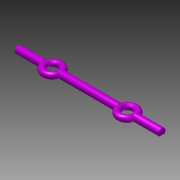
# Autodesk Inventor part: new string management system
Saved by Autodesk Inventor 2013 (Build 170138000, 138)
## iProperties
Created: 2014-03-08
Part Number: new string management system
Material: ABS Plastic
Document SubType Name: Modeling
Designer: kahohbein
Density: 1 g/cm^3
Author: kahohbein
Autodesk Inventor part; units mm, degrees
ref_plane "XZ Plane" through (0, 0, 0) normal (0, 1, 0) x (-1, 0, 0)
ref_plane "XY Plane" through (0, 0, 0) normal (0, 0, 1) x (1, 0, 0)
sketch "Sketch1" plane through (0, 0, 0) normal (0, 0, 1) x (1, 0, 0)
  line L0 (0, 0) -> (0, 6.5228)
  circle A0 centre (5, 0) radius 2
  dimension "d0" = 4
  dimension "d1" = 5
  constraints: 2 end point, 1 centre point, 1 vertical
  measures "d0" diameter of A0
  measures "d1" distance from line of A0.centre L0
revolve "Revolution1" add sketch "Sketch1" angle 360 about axis through (0, 0, 0) along (0, 1, 0)
ref_plane "Work Plane1" through (5.3, 0, 0) normal (1, 0, 0) x (0, 1, 0)
sketch "Sketch2" plane through (5.3, 0, 0) normal (1, 0, 0) x (0, 1, 0)
  circle A0 centre (0, 0) radius 2.3241
  dimension "d4" = 4.6482
  constraints: 1 centre point, 1 coincident
  measures "d4" diameter of A0
extrude "Extrusion1" add sketch "Sketch2" along normal blind 17.145
pattern_of_nothing "Mirror1"
sketch "Sketch3" plane through (-5.3, 0, 0) normal (-1, 0, 0) x (0, 1, 0)
  circle A0 centre (0, 0) radius 2.3241
  dimension "d7" = 4.6482
  constraints: 1 centre point, 1 coincident
  measures "d7" diameter of A0
extrude "Extrusion2" add sketch "Sketch3" along normal blind 19.05
mirror "Mirror2" about plane through (-24.35, 0, 0) normal (-1, 0, 0) of "Extrusion1", "Revolution1", "Extrusion2"
ref_plane "Work Plane5" through (0, -1.5875, 0) normal (0, -1, 0) x (1, 0, 0)
ref_plane "Work Plane4" through (0, 0, 0) normal (0, -1, 0) x (1, 0, 0)
sketch "Sketch4" plane through (0, -1.5875, 0) normal (0, -1, 0) x (1, 0, 0)
  line L0 (27.3527, -8.2733) -> (-72.0962, -8.2733)
  line L1 (-72.0962, -8.2733) -> (-72.0962, 10.4683)
  line L2 (-72.0962, 10.4683) -> (27.3527, 10.4683)
  line L3 (27.3527, 10.4683) -> (27.3527, -8.2733)
  point P0 (0, 0)
  constraints: 8 end point, 2 parallel, 1 horizontal, 1 perpendicular
extrude "Extrusion3" cut sketch "Sketch4" along normal blind 11.1125
ref_plane "Work Plane2" through (-5.3, 0, 0) normal (1, 0, 0) x (0, 1, 0)
body "Solid1"
